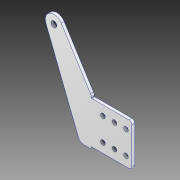
# Autodesk Inventor part: VersaChassis Bumper Support Plate
Saved by Autodesk Inventor 2023 (Build 270158000, 158)
## iProperties
Created: 2021-12-12
Part Number: VersaChassis Bumper Support Plate
Material: Aluminum 6061
Document SubType Name: Modeling
Density: 2.7 g/cm^3
Appearance: Aluminum - Flat
Appearance: Aluminum - Dark
Mass: 45.2618 g
Surface Area: 121.913 cm^2
Volume: 16.7636 cm^3
Mass: 55.6267 g
Surface Area: 149.196 cm^2
Volume: 20.6025 cm^3
Mass: 51.4818 g
Surface Area: 138.042 cm^2
Volume: 19.0673 cm^3
Autodesk Inventor part; units mm, degrees
ref_plane "YZ Plane" through (0, 0, 0) normal (1, 0, 0) x (0, 1, 0)
ref_plane "XZ Plane" through (0, 0, 0) normal (0, 1, 0) x (-1, 0, 0)
ref_plane "XY Plane" through (0, 0, 0) normal (0, 0, 1) x (1, 0, 0)
sketch "Sketch1" plane through (0, 0, 0) normal (0, 0, 1) x (1, 0, 0)
  arc A0 (8.0581, 5.0787) -> (-8.8609, -3.4943) centre (0, 0) ccw
  line L0 (8.0581, 5.0787) -> (41.275, -47.625)
  line L1 (41.275, -47.625) -> (41.275, -49.911)
  line L2 (41.275, -49.911) -> (85.725, -49.911)
  line L3 (85.725, -49.911) -> (85.725, -96.139)
  line L4 (28.575, -98.425) -> (-8.8609, -3.4943)
  circle A1 centre (0, 0) radius 3.2512
  line L5 (85.725, -96.139) -> (41.275, -96.139)
  line L6 (41.275, -96.139) -> (41.275, -98.425)
  line L7 (41.275, -98.425) -> (28.575, -98.425)
  line L8 (85.725, -73.025) -> (85.7238, -73.025) construction
  circle A2 centre (79.375, -60.325) radius 2.4892
  circle A3 centre (66.675, -60.325) radius 2.4892
  circle A4 centre (79.375, -85.725) radius 2.4892
  circle A5 centre (66.675, -85.725) radius 2.4892
  circle A6 centre (53.975, -60.325) radius 2.4892
  circle A7 centre (53.975, -85.725) radius 2.4892
  line L9 (-9.525, 139.734) -> (-9.525, 40.2644) construction
  line L10 (-53.9331, -9.525) -> (112.0207, -9.525) construction
  dimension "d0" = 19.05
  dimension "d1" = 6.5024
  dimension "d2" = 2.286
  dimension "d3" = 4.9784
  dimension "d6" = 12.7
  dimension "d9" = 25.4
  dimension "d12" = 12.7
  dimension "d13" = 50.8
  dimension "d14" = 6.35
  dimension "d15" = 12.7
  dimension "d16" = 50.8
  dimension "d17" = 12.7
  dimension "d18" = 38.1
  constraints: 22 end point, 8 centre point, 4 horizontal, 4 perpendicular, 4 tangent, 3 vertical, 2 coincident, 2 collinear, 2 point on circle, 1 midpoint, 10 other
  measures "d0" diameter of A0
  measures "d1" diameter of A1
  measures "d2" distance of L0.end L1.end
  measures "d3" diameter of A2
  measures "d6" distance of A2.centre A3.centre
  measures "d9" distance of A2.centre A4.centre
  measures "d12" distance from line of L8 A2.centre
  measures "d13" distance between parallel lines of L1 L9
  measures "d14" distance from line of L3 A2.centre
  measures "d15" distance of L6.end L4.start
  measures "d16" distance of L6.end L0.end
  measures "d17" horizontal distance of L1.end A6.centre
  measures "d18" distance from line of L10 L0.end
extrude "Extrusion1" add sketch "Sketch1" along normal blind 3.175
fillet "Fillet1" radius 3.175 2 edges at (85.725, -49.911, 1.5875) (85.725, -96.139, 1.5875)
fillet "Fillet1" radius 6.35 2 edges at (28.575, -98.425, 1.5875) (41.275, -47.625, 1.5875)
fillet "Fillet1" radius 1.5875 1 edges at (41.275, -98.425, 1.5875)
body "Solid1"
